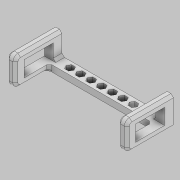
# Autodesk Inventor part: Chassis_atras_V4
Saved by Autodesk Inventor 2022.2 (Build 262287010, 287A)
## iProperties
Created: 2022-06-14
Part Number: Chassis_atras_V4
Material: Genérico
Document SubType Name: Modeling
Designer: Usuario
Density: 1 g/cm^3
Appearance: Valor por defecto
Author: Usuario
Autodesk Inventor part; units mm, degrees
ref_plane "YZ Plane" through (0, 0, 0) normal (1, 0, 0) x (0, 1, 0)
ref_plane "XZ Plane" through (0, 0, 0) normal (0, 1, 0) x (-1, 0, 0)
ref_plane "XY Plane" through (0, 0, 0) normal (0, 0, 1) x (1, 0, 0)
sketch "Boceto1" plane through (0, 0, 0) normal (0, 1, 0) x (-1, 0, 0)
  line L0 (29.505, -15) -> (44.5466, 0) construction
  line L1 (33.6552, -19.1617) -> (29.505, -15) construction
  line L2 (0, 0) -> (0, 6.3504) construction
  line L3 (0, 0) -> (0, -23.2363) construction
  line L4 (0, -15) -> (29.505, -15)
  line L5 (47.8008, -25) -> (47.8008, 12)
  line L6 (47.8008, 12) -> (40.8008, 12)
  line L7 (40.8008, 12) -> (40.8008, -15)
  line L8 (40.8008, -15) -> (29.505, -15)
  line L9 (47.8008, -25) -> (0, -25)
  line L10 (0, -15) -> (-29.505, -15)
  line L11 (-47.8008, -25) -> (-47.8008, 12)
  line L12 (-47.8008, 12) -> (-40.8008, 12)
  line L13 (-40.8008, 12) -> (-40.8008, -15)
  line L14 (-40.8008, -15) -> (-29.505, -15)
  line L15 (-47.8008, -25) -> (0, -25)
  dimension "d70" = 7
  dimension "d71" = 37
  constraints: 32 end point, 5 symmetric about line, 3 horizontal, 3 vertical, 2 perpendicular, 1 point on line
  measures "d70" distance of L5.end L6.end
  measures "d71" distance of L5.start L5.end
extrude "Extrusión1" add sketch "Boceto1" along normal blind 5
sketch "Boceto2" plane through (0, 5, 0) normal (0, 1, 0) x (1, 0, 0)
  line L0 (-2.6123, 17.25) -> (-5.7877, 17.25)
  line L1 (-5.7877, 17.25) -> (-7.3754, 20)
  line L2 (-7.3754, 20) -> (-5.7877, 22.75)
  line L3 (-5.7877, 22.75) -> (-2.6123, 22.75)
  line L4 (-2.6123, 22.75) -> (-1.0246, 20)
  line L5 (-1.0246, 20) -> (-2.6123, 17.25)
  line L6 (21.3433, 15) -> (-21.3433, 15) projected
  line L7 (-14.1877, 22.75) -> (-11.0123, 22.75)
  line L8 (-15.7754, 20) -> (-14.1877, 22.75)
  line L9 (-14.1877, 17.25) -> (-15.7754, 20)
  line L10 (-11.0123, 17.25) -> (-14.1877, 17.25)
  line L11 (-9.4246, 20) -> (-11.0123, 17.25)
  line L12 (-11.0123, 22.75) -> (-9.4246, 20)
  line L13 (-22.5877, 22.75) -> (-19.4123, 22.75)
  line L14 (-24.1754, 20) -> (-22.5877, 22.75)
  line L15 (-22.5877, 17.25) -> (-24.1754, 20)
  line L16 (-19.4123, 17.25) -> (-22.5877, 17.25)
  line L17 (-17.8246, 20) -> (-19.4123, 17.25)
  line L18 (-19.4123, 22.75) -> (-17.8246, 20)
  line L19 (-30.9877, 22.75) -> (-27.8123, 22.75)
  line L20 (-32.5754, 20) -> (-30.9877, 22.75)
  line L21 (-30.9877, 17.25) -> (-32.5754, 20)
  line L22 (-27.8123, 17.25) -> (-30.9877, 17.25)
  line L23 (-26.2246, 20) -> (-27.8123, 17.25)
  line L24 (-27.8123, 22.75) -> (-26.2246, 20)
  line L25 (2.6123, 17.25) -> (5.7877, 17.25)
  line L26 (5.7877, 17.25) -> (7.3754, 20)
  line L27 (7.3754, 20) -> (5.7877, 22.75)
  line L28 (5.7877, 22.75) -> (2.6123, 22.75)
  line L29 (2.6123, 22.75) -> (1.0246, 20)
  line L30 (1.0246, 20) -> (2.6123, 17.25)
  line L31 (14.1877, 22.75) -> (11.0123, 22.75)
  line L32 (15.7754, 20) -> (14.1877, 22.75)
  line L33 (14.1877, 17.25) -> (15.7754, 20)
  line L34 (11.0123, 17.25) -> (14.1877, 17.25)
  line L35 (9.4246, 20) -> (11.0123, 17.25)
  line L36 (11.0123, 22.75) -> (9.4246, 20)
  line L37 (22.5877, 22.75) -> (19.4123, 22.75)
  line L38 (24.1754, 20) -> (22.5877, 22.75)
  line L39 (22.5877, 17.25) -> (24.1754, 20)
  line L40 (19.4123, 17.25) -> (22.5877, 17.25)
  line L41 (17.8246, 20) -> (19.4123, 17.25)
  line L42 (19.4123, 22.75) -> (17.8246, 20)
  line L43 (30.9877, 22.75) -> (27.8123, 22.75)
  line L44 (32.5754, 20) -> (30.9877, 22.75)
  line L45 (30.9877, 17.25) -> (32.5754, 20)
  line L46 (27.8123, 17.25) -> (30.9877, 17.25)
  line L47 (26.2246, 20) -> (27.8123, 17.25)
  line L48 (27.8123, 22.75) -> (26.2246, 20)
  point P0 (0, 0)
  point P1 (-4.2, 20)
  point P2 (0, 0)
  point P3 (4.2, 20)
  dimension "d17" = 5.5
  dimension "d22" = 8.4
  constraints: 96 end point, 2 horizontal, 49 other
  measures "d17" distance between parallel lines of L0 L3
  measures "d22" distance of L2.end L7.start
extrude "Extrusión2" cut sketch "Boceto2" against normal up to surface (5 mm away)
sketch "Boceto11" plane through (0, 5, 0) normal (0, 1, 0) x (1, 0, 0)
  line L0 (-47.8008, -12) -> (-40.8008, -12) projected
  line L1 (47.8008, 25) -> (-47.8008, 25) projected
  line L2 (-47.8008, -12) -> (-40.8008, -12)
  line L3 (-40.8008, -12) -> (-40.8008, 25)
  line L4 (-40.8008, 25) -> (-47.8008, 25)
  line L5 (-47.8008, 25) -> (-47.8008, -12)
  line L6 (0, 0) -> (0, -8.2135) construction
  line L7 (47.8008, -12) -> (40.8008, -12)
  line L8 (40.8008, -12) -> (40.8008, 25)
  line L9 (40.8008, 25) -> (47.8008, 25)
  line L10 (47.8008, 25) -> (47.8008, -12)
  constraints: 18 end point, 6 symmetric about line, 2 parallel, 1 horizontal, 1 perpendicular, 1 point on line, 1 vertical
extrude "Extrusión7" add sketch "Boceto11" along normal blind 17.5
sketch "Boceto12" plane through (47.8008, 0, 12) normal (1, 0, 0) x (0, 0, -1)
  line L0 (7, 17.5) -> (30, 17.5)
  line L1 (30, 17.5) -> (30, 5)
  line L2 (30, 5) -> (7, 5)
  line L3 (7, 5) -> (7, 17.5)
  line L4 (37, 22.5) -> (0, 22.5) projected
  line L5 (18.5, 22.5) -> (18.5, 29.9213) construction
  line L6 (0, 0) -> (0, 22.5) projected
  line L7 (0, 11.25) -> (-3.0724, 11.25) construction
  point P0 (12, 0)
  dimension "d74" = 12.5
  dimension "d75" = 23
  constraints: 12 end point, 2 horizontal, 2 midpoint, 2 parallel, 2 symmetric about line, 1 perpendicular, 1 vertical
  measures "d74" distance of L0.end L1.end
  measures "d75" distance of L1.end L2.end
extrude "Extrusión8" cut sketch "Boceto12" against normal through all
fillet "Empalme5" radius 4 4 edges at (-44.3008, 0, 12) (-44.3008, 22.5, 12) (44.3008, 0, 12) (44.3008, 22.5, 12)
chamfer "Chaflán3" distance 2 angle 45 20 edges at (47.8008, 22.5, -8.5) (47.8008, 21.3284, 10.8284) (47.8008, 11.25, 12) (47.8008, 1.1716, 10.8284) (47.8008, 0, -8.5) (-47.8008, 22.5, -8.5) (-47.8008, 21.3284, 10.8284) (-47.8008, 11.25, 12) (-47.8008, 1.1716, 10.8284) (-47.8008, 0, -8.5) (-40.8008, 22.5, -8.5) (-40.8008, 21.3284, 10.8284) (-40.8008, 11.25, 12) (-40.8008, 1.1716, 10.8284) (-40.8008, 0, -3.5) (40.8008, 22.5, -8.5) (40.8008, 21.3284, 10.8284) (40.8008, 11.25, 12) (40.8008, 1.1716, 10.8284) (40.8008, 0, -3.5)
chamfer "Chaflán4" distance 2 angle 45 6 edges at (-40.8008, 5, -21.5) (40.8008, 5, -21.5) (-40.8008, 3.5, -15) (-41.8008, 1, -15) (41.8008, 1, -15) (40.8008, 3.5, -15)
